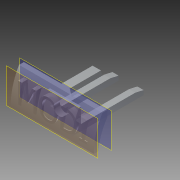
# Autodesk Inventor part: logo
Saved by Autodesk Inventor 2013 (Build 170138000, 138)
## iProperties
Created: 2013-06-03
Part Number: logo
Material: Glass
Document SubType Name: Modeling
Designer: otrab
Density: 1 g/cm^3
Author: otrab
Autodesk Inventor part; units mm, degrees
ref_plane "YZ Plane" through (0, 0, 0) normal (1, 0, 0) x (0, 1, 0)
ref_plane "XY Plane" through (0, 0, 0) normal (0, 0, 1) x (1, 0, 0)
sketch "Sketch1" plane through (0, 0, 0) normal (1, 0, 0) x (0, 1, 0)
  arc A0 (0, 0) -> (-4.3568, -15) centre (23.6432, -15) ccw
  arc A1 (-2.3376, 0) -> (-6.3568, -15) centre (23.6432, -15) ccw
  line L0 (0, 0) -> (-2.3376, 0)
  line L1 (0, 0) -> (0, -15) construction
  line L2 (-4.3568, -15) -> (-6.3568, -15)
  dimension "d1" = 28
  dimension "d2" = 2
  dimension "d5" = 15
  constraints: 6 end point, 4 point on circle, 2 centre point, 1 coincident, 1 horizontal
  measures "d1" radius of A0
  measures "d2" radial gap between concentric circles of A1 A0
  measures "d5" distance of L0.start L1.end
extrude "Extrusion1" add sketch "Sketch1" along normal blind 40
ref_plane "Work Plane1" through (0, 0, 0) normal (0, 1, 0) x (-1, 0, 0)
sketch "Sketch2" plane through (0, 0, 0) normal (0, 1, 0) x (-1, 0, 0)
  line L0 (-27.4711, -15) -> (-24.4711, -15)
  line L1 (-24.4711, -15) -> (-24.4711, -12)
  line L2 (-24.4711, -12) -> (-27.4711, -12)
  line L3 (-27.4711, -12) -> (-27.4711, -15)
  line L4 (-12.5289, -15) -> (-15.5289, -15)
  line L5 (-15.5289, -15) -> (-15.5289, -12)
  line L6 (-15.5289, -12) -> (-12.5289, -12)
  line L7 (-12.5289, -12) -> (-12.5289, -15)
  line L8 (0, 0) -> (-20, 0) construction
  line L9 (-20, 0) -> (-18, 0)
  line L10 (-20, 0) -> (-20, -3) construction
  line L11 (-20, -3) -> (-17, -3)
  line L12 (-17, -3) -> (-18, 0)
  line L13 (-40, 0) -> (-20, 0) construction
  line L14 (-20, 0) -> (-22, 0)
  line L15 (-20, -3) -> (-23, -3)
  line L16 (-23, -3) -> (-22, 0)
  point P0 (-20, -15)
  dimension "d35" = 20
  dimension "d36" = 2
  dimension "d37" = 3
  dimension "d38" = 3
  constraints: 34 end point, 3 symmetric about line, 2 perpendicular, 2 point on line, 1 parallel
  measures "d35" distance of L8.start L8.end
  measures "d36" distance of L8.end L9.end
  measures "d37" distance of L8.end L10.end
  measures "d38" distance of L10.end L11.end
extrude "Extrusion2" add sketch "Sketch2" against normal up to surface round surface about axis through (0, 23.6432, -15) along (1, 0, 0) radius 28 far side no
sketch "Sketch3" plane through (0, 0, 0) normal (0, 1, 0) x (-1, 0, 0)
  line L0 (-20, -7.5) -> (-46.0081, -7.5) construction
  line L1 (-12.5, -15) -> (-15.5, -15)
  line L2 (-15.5, -15) -> (-15.5, -12)
  line L3 (-15.5, -12) -> (-12.5, -12)
  line L4 (-12.5, -12) -> (-12.5, -15)
  line L5 (-27.5, -15) -> (-24.5, -15)
  line L6 (-24.5, -15) -> (-24.5, -12)
  line L7 (-24.5, -12) -> (-27.5, -12)
  line L8 (-27.5, -12) -> (-27.5, -15)
  point P0 (0, 0)
  point P1 (-20, -15)
  constraints: 18 end point
extrude "Extrusion3" add sketch "Sketch3" along normal blind 30
sketch "Sketch4" plane through (27.5, 0, -12) normal (1, 0, 0) x (0, 0, -1)
  line L0 (0, 30) -> (3, 30) projected
  line L1 (0, 0) -> (0, 30) projected
  line L2 (0, 30) -> (0, 26)
  line L3 (0, 26) -> (0.9, 30)
  line L4 (0.9, 30) -> (0, 30)
  point P0 (-12, 0)
  dimension "d22" = 4
  dimension "d23" = 4.1
  constraints: 6 end point, 2 point on line, 1 perpendicular
  measures "d22" distance of L0.start L2.end
  measures "d23" distance of L2.end L3.end
extrude "Extrusion4" cut sketch "Sketch4" against normal up to surface (15 mm away)
ref_plane "Work Plane2" through (0, -6.5, 0) normal (0, -1, 0) x (1, 0, 0)
sketch "Sketch5" plane through (0, -6.5, 0) normal (0, -1, 0) x (1, 0, 0)
  line L0 (2.7031, -2.3909) -> (34.0135, -2.3909) construction
  line L1 (34.0135, -2.3909) -> (34.0135, -11.7702) construction
  line L2 (34.0135, -11.7702) -> (2.7031, -11.7702) construction
  line L3 (2.7031, -11.7702) -> (2.7031, -2.3909) construction
  line L4 (12.2898, -12.6016) -> (10.9608, -12.6016)
  line L5 (10.9608, -12.6016) -> (10.9608, -3.9873)
  line L6 (10.9608, -3.9873) -> (8.3514, -9.8463)
  line L7 (8.3514, -9.8463) -> (7.541, -9.8463)
  line L8 (7.541, -9.8463) -> (4.9559, -3.9873)
  line L9 (4.9559, -3.9873) -> (4.9559, -12.6016)
  line L10 (4.9559, -12.6016) -> (3.7161, -12.6016)
  line L11 (3.7161, -12.6016) -> (3.7161, -2.6016)
  line L12 (3.7161, -2.6016) -> (5.5313, -2.6016)
  line L13 (5.5313, -2.6016) -> (8.0272, -8.1689)
  line L14 (8.0272, -8.1689) -> (10.4422, -2.6016)
  line L15 (10.4422, -2.6016) -> (12.2898, -2.6016)
  line L16 (12.2898, -2.6016) -> (12.2898, -12.6016)
  spline S0 degree 2 poles (21.3903, -3.7442) (21.9576, -4.4087) (22.5896, -6.3536) (22.5896, -7.6016) knots 0 0 0 1 2 2 2
  spline S1 degree 2 poles (22.5896, -7.6016) (22.5896, -8.8172) (21.9738, -10.7864) (21.3903, -11.4509) knots 0 0 0 1 2 2 2
  spline S2 degree 2 poles (21.3903, -11.4509) (20.7744, -12.1478) (19.1456, -12.8123) (18.165, -12.8123) knots 0 0 0 1 2 2 2
  spline S3 degree 2 poles (18.165, -12.8123) (17.152, -12.8123) (15.5313, -12.1235) (14.9397, -11.4509) knots 0 0 0 1 2 2 2
  spline S4 degree 2 poles (14.9397, -11.4509) (14.3644, -10.7864) (13.7485, -8.8334) (13.7485, -7.6016) knots 0 0 0 1 2 2 2
  spline S5 degree 2 poles (13.7485, -7.6016) (13.7485, -6.3455) (14.3725, -4.4331) (14.9478, -3.7442) knots 0 0 0 1 2 2 2
  spline S6 degree 2 poles (14.9478, -3.7442) (15.5313, -3.0797) (17.1601, -2.3909) (18.165, -2.3909) knots 0 0 0 1 2 2 2
  spline S7 degree 2 poles (18.165, -2.3909) (19.1861, -2.3909) (20.823, -3.104) (21.3903, -3.7442) knots 0 0 0 1 2 2 2
  spline S8 degree 2 poles (21.2039, -7.6016) (21.2039, -6.613) (20.7744, -5.0814) (20.3854, -4.5789) knots 0 0 0 1 2 2 2
  spline S9 degree 2 poles (20.3854, -4.5789) (19.9883, -4.0603) (18.87, -3.5416) (18.1731, -3.5416) knots 0 0 0 1 2 2 2
  spline S10 degree 2 poles (18.1731, -3.5416) (17.4519, -3.5416) (16.366, -4.0441) (15.9527, -4.5789) knots 0 0 0 1 2 2 2
  spline S11 degree 2 poles (15.9527, -4.5789) (15.5556, -5.0895) (15.1342, -6.6292) (15.1342, -7.6016) knots 0 0 0 1 2 2 2
  spline S12 degree 2 poles (15.1342, -7.6016) (15.1342, -9.5708) (16.7874, -11.6616) (18.1731, -11.6616) knots 0 0 0 1 2 2 2
  spline S13 degree 2 poles (18.1731, -11.6616) (19.5588, -11.6616) (21.2039, -9.5708) (21.2039, -7.6016) knots 0 0 0 1 2 2 2
  spline S14 degree 2 poles (31.9332, -7.6097) (31.9332, -8.9792) (30.823, -11.1835) (29.8911, -11.7993) knots 0 0 0 1 2 2 2
  spline S15 degree 2 poles (29.8911, -11.7993) (29.1294, -12.2775) (27.5653, -12.6016) (26.3498, -12.6016) knots 0 0 0 1 2 2 2
  line L17 (26.3498, -12.6016) -> (24.0483, -12.6016)
  line L18 (24.0483, -12.6016) -> (24.0483, -2.6016)
  line L19 (24.0483, -2.6016) -> (26.3255, -2.6016)
  spline S16 degree 2 poles (26.3255, -2.6016) (27.7355, -2.6016) (29.34, -3.023) (29.9073, -3.3958) knots 0 0 0 1 2 2 2
  spline S17 degree 2 poles (29.9073, -3.3958) (30.8717, -4.036) (31.9332, -6.151) (31.9332, -7.6097) knots 0 0 0 1 2 2 2
  spline S18 degree 2 poles (30.5475, -7.5935) (30.5475, -6.4428) (29.7858, -4.8139) (29.0321, -4.352) knots 0 0 0 1 2 2 2
  spline S19 degree 2 poles (29.0321, -4.352) (28.4973, -4.036) (27.2898, -3.7523) (26.3903, -3.7523) knots 0 0 0 1 2 2 2
  line L20 (26.3903, -3.7523) -> (25.3773, -3.7523)
  line L21 (25.3773, -3.7523) -> (25.3773, -11.4509)
  line L22 (25.3773, -11.4509) -> (26.3903, -11.4509)
  spline S20 degree 2 poles (26.3903, -11.4509) (27.2736, -11.4509) (28.6107, -11.1673) (29.1537, -10.7864) knots 0 0 0 1 2 2 2
  spline S21 degree 2 poles (29.1537, -10.7864) (29.8506, -10.3164) (30.5475, -8.7604) (30.5475, -7.5935) knots 0 0 0 1 2 2 2
  line L23 (36.8603, -12.6016) -> (32.9867, -12.6016)
  line L24 (32.9867, -12.6016) -> (32.9867, -11.5805)
  line L25 (32.9867, -11.5805) -> (34.259, -11.5805)
  line L26 (34.259, -11.5805) -> (34.259, -3.6227)
  line L27 (34.259, -3.6227) -> (32.9867, -3.6227)
  line L28 (32.9867, -3.6227) -> (32.9867, -2.6016)
  line L29 (32.9867, -2.6016) -> (36.8603, -2.6016)
  line L30 (36.8603, -2.6016) -> (36.8603, -3.6227)
  line L31 (36.8603, -3.6227) -> (35.588, -3.6227)
  line L32 (35.588, -3.6227) -> (35.588, -11.5805)
  line L33 (35.588, -11.5805) -> (36.8603, -11.5805)
  line L34 (36.8603, -11.5805) -> (36.8603, -12.6016)
  point P0 (0, 0)
  constraints: 2 other
extrude "Extrusion5" add sketch "Sketch5" against normal up to surface round surface about axis through (0, 23.6432, -15) along (1, 0, 0) radius 30 far side no
sketch "Sketch6" plane through (0, 0, 0) normal (0, 1, 0) x (1, 0, 0)
  line L0 (24.5, 12) -> (24.4711, 12) projected
  line L1 (18.003, 0) -> (16.9798, 2.9998)
  line L2 (16.9798, 2.9998) -> (22.9798, 2.9998)
  line L3 (22.9798, 2.9998) -> (22.003, 0)
  line L4 (22.003, 0) -> (18.003, 0)
  point P0 (0, 0)
  dimension "d39" = 6
  dimension "d40" = 4
  constraints: 8 end point, 2 parallel
  measures "d39" distance of L1.end L2.end
  measures "d40" distance of L3.end L1.start
extrude "Extrusion6" add sketch "Sketch6" along normal blind 15
sketch "Sketch7" plane through (40, 0, 0) normal (1, 0, 0) x (0, 0, -1)
  arc A0 (0, 0) -> (15, -4.3568) centre (15, 23.6432) ccw projected
  line L0 (15, -6.3568) -> (15, -4.3568) projected
  line L1 (0, 0) -> (3, 0)
  arc A1 (3, 0) -> (15, -4.3568) centre (18.304, 23.4476) ccw
  dimension "d41" = 3
  dimension "d42" = 28
  constraints: 3 point on circle, 2 end point, 1 centre point, 1 perpendicular
  measures "d41" distance of L1.start L1.end
  measures "d42" radius of A1
extrude "Extrusion7" add sketch "Sketch7" against normal up to surface (40 mm away)
sketch "Sketch10" plane through (0, 0, 0) normal (0, 1, 0) x (-1, 0, 0)
  line L0 (-27.5, -12) -> (-12.5, -12)
  line L1 (-12.5, -12) -> (-12.5, -4.6566)
  line L2 (-12.5, -4.6566) -> (-27.5, -4.6566)
  line L3 (-27.5, -4.6566) -> (-27.5, -12)
  point P0 (0, 0)
  point P1 (-24.5, -12)
  constraints: 8 end point, 2 parallel, 1 horizontal, 1 perpendicular
extrude "Extrusion8" add sketch "Sketch10" against normal up to next
sketch "Sketch11" plane through (0, 0, 0) normal (0, 1, 0) x (1, 0, 0)
  circle A0 centre (20, 8.3283) radius 2.75
  point P0 (0, 0)
  dimension "d47" = 5.5
  constraints: 1 centre point, 1 other
  measures "d47" diameter of A0
extrude "Extrusion9" cut sketch "Sketch11" against normal blind 3 draft -0.5
body "Solid1"
